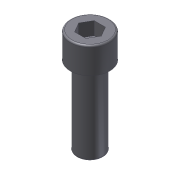
# Autodesk Inventor part: Bolt_0.25_20_0.75len_SocketHead
Saved by Autodesk Inventor 2012 (Build 160160000, 160)
## iProperties
Created: 2013-02-01
Part Number: Bolt_0.25_20_0.75len_SocketHead
Material: Stainless Steel, Austenitic
Document SubType Name: Modeling
Designer: JesseK
Density: 8.03 g/cm^3
Mass: 7.96939 g
Surface Area: 7.52974 cm^2
Volume: 0.992452 cm^3
Author: JesseK
Autodesk Inventor part; units mm, degrees
ref_plane "YZ Plane" through (0, 0, 0) normal (1, 0, 0) x (0, 1, 0)
ref_plane "XZ Plane" through (0, 0, 0) normal (0, 1, 0) x (-1, 0, 0)
ref_plane "XY Plane" through (0, 0, 0) normal (0, 0, 1) x (1, 0, 0)
sketch "Sketch1" plane through (0, 0, 0) normal (0, 1, 0) x (-1, 0, 0)
  circle A0 centre (0, 0) radius 3.175
  dimension "d0" = 6.35
  constraints: 1 centre point, 1 coincident
  measures "d0" diameter of A0
extrude "Extrusion1" add sketch "Sketch1" along normal blind 19.05
sketch "Sketch2" plane through (0, 19.05, 0) normal (0, 1, 0) x (1, 0, 0)
  circle A0 centre (0, 0) radius 3.175 projected
  circle A1 centre (0, 0) radius 4.7625
  dimension "d3" = 9.525
  constraints: 1 centre point, 1 coincident
  measures "d3" diameter of A1
extrude "Extrusion2" add sketch "Sketch2" along normal blind 6.35 contours A0 | A1
sketch "Sketch3" plane through (0, 25.4, 0) normal (0, 1, 0) x (1, 0, 0)
  circle A0 centre (0, 0) radius 4.7625 projected
  line L0 (-1.3748, 2.3812) -> (1.3748, 2.3813)
  line L1 (1.3748, 2.3813) -> (2.7496, 0)
  line L2 (2.7496, 0) -> (1.3748, -2.3813)
  line L3 (1.3748, -2.3813) -> (-1.3748, -2.3813)
  line L4 (-1.3748, -2.3813) -> (-2.7496, 0)
  line L5 (-2.7496, 0) -> (-1.3748, 2.3812)
  dimension "d6" = 4.7625
  constraints: 12 end point, 1 coincident, 1 horizontal, 13 other
  measures "d6" distance between parallel lines of L3 L0
extrude "Extrusion3" cut sketch "Sketch3" against normal blind 3.175 contours L0 L1 L2 L3 L4 L5
fillet "Fillet1" radius 0.3969 3 edges at (3.175, 19.05, 0) (-4.7625, 25.4, 0) (3.175, 0, 0)
body "Solid1"
